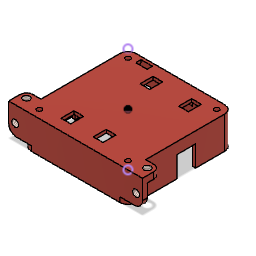
Com Top A (Autodesk Fusion 360 design; units mm, degrees)
Autodesk Fusion 360 part; units mm, degrees
sketch "Sketch17" plane through (0, 0, 0) normal (0, 1, 0) x (1, 0, 0)
  line L0 (-32.5, 32.5) -> (32.5, 32.5)
  line L1 (32.5, 32.5) -> (32.5, -32.5)
  line L2 (32.5, -32.5) -> (-32.5, -32.5)
  line L3 (-32.5, -32.5) -> (-32.5, 32.5)
  line L4 (-32.5, 32.5) -> (32.5, -32.5) construction
  line L5 (32.5, 32.5) -> (-32.5, -32.5) construction
  dimension "d63" = 65
  dimension "d64" = 65
  constraint horizontal L0
  constraint perpendicular L0 L1
  constraint parallel L0 L2
  constraint parallel L1 L3
  constraint coincident L4 origin
  constraint coincident L5 origin
  measures "d63" distance of L1.end L2.end
  measures "d64" distance of L0.end L1.end
extrude "Extrude19" add sketch "Sketch17" along normal blind 2 makes body 1
sketch "Sketch18" plane through (0, 2, 0) normal (0, 1, 0) x (-1, 0, 0)
  line L0 (-32.5, 32.5) -> (-32.5, -32.5)
  line L1 (-32.5, -32.5) -> (32.5, -32.5)
sketch "Sketch20" plane through (0, 0, 0) normal (0, -1, 0) x (1, 0, 0)
  line L0 (32.5, 32.5) -> (-32.5, 32.5)
  line L1 (-32.5, 32.5) -> (-32.5, -32.5)
  line L2 (-32.5, -32.5) -> (32.5, -32.5)
  line L3 (32.5, -32.5) -> (32.5, 32.5)
  line L4 (30.75, -30.75) -> (-30.75, -30.75)
  line L5 (-30.75, -30.75) -> (-30.75, 30.75)
  line L6 (-30.75, 30.75) -> (30.75, 30.75)
  line L7 (30.75, 30.75) -> (30.75, -30.75)
  line L8 (30.75, -30.75) -> (-30.75, 30.75) construction
  line L9 (-30.75, -30.75) -> (30.75, 30.75) construction
  line L10 (-32.5, 22.7576) -> (-30.75, 22.7576)
  line L11 (-30.75, 22.7576) -> (-30.75, 2.2148)
  line L12 (-30.75, 2.2148) -> (-32.5, 2.2148)
  line L13 (-32.5, 2.2148) -> (-32.5, 22.7576)
  line L14 (-32.5, -3.5662) -> (-30.75, -3.5662)
  line L15 (-30.75, -3.5662) -> (-30.75, -14.3569)
  line L16 (-30.75, -14.3569) -> (-32.5, -14.3569)
  line L17 (-32.5, -14.3569) -> (-32.5, -3.5662)
  line L18 (-22.4493, -30.75) -> (-15.7732, -30.75)
  line L19 (-15.7732, -30.75) -> (-15.7732, -32.5)
  line L20 (-15.7732, -32.5) -> (-22.4493, -32.5)
  line L21 (-22.4493, -32.5) -> (-22.4493, -30.75)
  line L22 (-3.0358, -30.75) -> (9.2826, -30.75)
  line L23 (9.2826, -30.75) -> (9.2826, -32.5)
  line L24 (9.2826, -32.5) -> (-3.0358, -32.5)
  line L25 (-3.0358, -32.5) -> (-3.0358, -30.75)
  line L26 (30.75, 1.1041) -> (32.5, 1.1041)
  line L27 (32.5, 1.1041) -> (32.5, -8.4005)
  line L28 (32.5, -8.4005) -> (30.75, -8.4005)
  line L29 (30.75, -8.4005) -> (30.75, 1.1041)
  dimension "d69" = 61.5
  dimension "d70" = 61.5
  constraint horizontal L4
  constraint perpendicular L4 L5
  constraint parallel L4 L6
  constraint parallel L5 L7
  constraint coincident L8 origin
  constraint coincident L9 origin
  constraint horizontal L10
  constraint vertical L11
  constraint horizontal L12
  constraint vertical L13
  constraint coincident L5 L11.end
  constraint coincident L1 L10.start
  constraint horizontal L14
  constraint vertical L15
  constraint horizontal L16
  constraint vertical L17
  constraint coincident L5 L15.end
  constraint coincident L1 L14.start
  constraint horizontal L18
  constraint vertical L19
  constraint horizontal L20
  constraint vertical L21
  constraint coincident L2 L19.end
  constraint coincident L4 L18.start
  constraint horizontal L22
  constraint vertical L23
  constraint horizontal L24
  constraint vertical L25
  constraint coincident L2 L23.end
  constraint coincident L4 L22.start
  constraint horizontal L26
  constraint vertical L27
  constraint horizontal L28
  constraint vertical L29
  constraint coincident L3 L27.end
  constraint coincident L7 L26.start
  measures "d69" distance of L5.end L6.end
  measures "d70" distance of L4.end L5.end
extrude "Extrude20" add sketch "Sketch20" along normal blind 25 contours L0 L1 L3 L5 L6 L7 L10 L26 | L2 L3 L4 L7 L23 L28 | L1 L5 L12 L14 | L1 L2 L4 L5 L16 L21 | L2 L4 L19 L25 bodies 1
extrude "Extrude21" add 1 faces at (32.5, -7.6667, 22.0347) along direction (1, 0, 0) blind 1 on bodies 1 bodies 1
extrude "Extrude22" add 1 faces at (25.4275, -7.6667, -32.5) along direction (0, 0, -1) blind 1 on bodies 1 bodies 1
extrude "Extrude23" add 1 faces at (-32.5, -7.6667, -27.119) along direction (-1, 0, 0) blind 1 on bodies 1 bodies 1
extrude "Extrude24" add 1 faces at (11.1667, -16, 32.5) along direction (0, 0, 1) blind 1 on bodies 1 bodies 1
sketch "Sketch21" plane through (0, 0, 0) normal (0, -1, 0) x (1, 0, 0)
  line L0 (-15.7732, -33.5) -> (-15.7732, -30.75)
  line L1 (-15.7732, -30.75) -> (-3.0358, -30.75)
  line L2 (-3.0358, -30.75) -> (-3.0358, -33.5)
  line L3 (-3.0358, -33.5) -> (9.2826, -33.5)
  line L4 (9.2826, -33.5) -> (9.2826, -30.75)
  line L5 (9.2826, -30.75) -> (30.75, -30.75)
  line L6 (30.75, -30.75) -> (30.75, -8.4005)
  line L7 (30.75, -8.4005) -> (33.5, -8.4005)
  line L8 (33.5, -8.4005) -> (33.5, 1.1041)
  line L9 (33.5, 1.1041) -> (30.75, 1.1041)
  line L10 (30.75, 1.1041) -> (30.75, 30.75)
  line L11 (30.75, 30.75) -> (-30.75, 30.75)
  line L12 (-30.75, 30.75) -> (-30.75, 22.7576)
  line L13 (-30.75, 22.7576) -> (-33.5, 22.7576)
  line L14 (-33.5, 22.7576) -> (-33.5, 2.2148)
  line L15 (-33.5, 2.2148) -> (-30.75, 2.2148)
  line L16 (-30.75, 2.2148) -> (-30.75, -3.5662)
  line L17 (-30.75, -3.5662) -> (-33.5, -3.5662)
  line L18 (-33.5, -3.5662) -> (-33.5, -14.3569)
  line L19 (-33.5, -14.3569) -> (-30.75, -14.3569)
  line L20 (-30.75, -14.3569) -> (-30.75, -30.75)
  line L21 (-30.75, -30.75) -> (-22.4493, -30.75)
  line L22 (-22.4493, -30.75) -> (-22.4493, -33.5)
  line L23 (-22.4493, -33.5) -> (-15.7732, -33.5)
  line L24 (30.75, -30.75) -> (-30.75, -30.75)
  line L25 (-30.75, -30.75) -> (-30.75, 30.75)
  line L26 (-30.75, 30.75) -> (30.75, 30.75)
  line L27 (30.75, 30.75) -> (30.75, -30.75)
  line L28 (30.75, -30.75) -> (-30.75, 30.75) construction
  line L29 (-30.75, -30.75) -> (30.75, 30.75) construction
  constraint horizontal L24
  constraint perpendicular L24 L25
  constraint parallel L24 L26
  constraint parallel L25 L27
  constraint coincident L28 origin
  constraint coincident L29 origin
  constraint coincident L5.end L6.start
extrude "Extrude25" add sketch "Sketch21" along normal blind 23 contours L0 L22 L23 L24 | L2 L3 L4 L24 | L17 L18 L19 L25 | L7 L8 L9 L27 | L13 L14 L15 L25 bodies 1
sketch "Sketch22" plane through (0, 0, 0) normal (0, -1, 0) x (1, 0, 0)
  line L0 (-30.75, -30.75) -> (30.75, -30.75)
  line L1 (30.75, -30.75) -> (30.75, 30.75)
  line L2 (30.75, 30.75) -> (-30.75, 30.75)
  line L3 (-30.75, 30.75) -> (-30.75, -30.75)
  line L4 (30.75, 30.75) -> (24.75, 30.75)
  line L5 (24.75, 30.75) -> (24.75, 24.75)
  line L6 (24.75, 24.75) -> (30.75, 24.75)
  line L7 (30.75, 24.75) -> (30.75, 30.75)
  line L8 (-30.75, 30.75) -> (-24.75, 30.75)
  line L9 (-24.75, 30.75) -> (-24.75, 24.75)
  line L10 (-24.75, 24.75) -> (-30.75, 24.75)
  line L11 (-30.75, 24.75) -> (-30.75, 30.75)
  line L12 (-30.75, -30.75) -> (-24.75, -30.75)
  line L13 (-24.75, -30.75) -> (-24.75, -24.75)
  line L14 (-24.75, -24.75) -> (-30.75, -24.75)
  line L15 (-30.75, -24.75) -> (-30.75, -30.75)
  line L16 (30.75, -30.75) -> (24.75, -30.75)
  line L17 (24.75, -30.75) -> (24.75, -24.75)
  line L18 (24.75, -24.75) -> (30.75, -24.75)
  line L19 (30.75, -24.75) -> (30.75, -30.75)
  dimension "d83" = 6
  dimension "d84" = 6
  dimension "d85" = 6
  dimension "d86" = 6
  dimension "d87" = 6
  dimension "d88" = 6
  dimension "d89" = 6
  dimension "d90" = 6
  constraint horizontal L4
  constraint vertical L5
  constraint horizontal L6
  constraint vertical L7
  constraint coincident L1.end L2.start
  constraint horizontal L8
  constraint vertical L9
  constraint horizontal L10
  constraint vertical L11
  constraint coincident L2.end L3.start
  constraint horizontal L12
  constraint vertical L13
  constraint horizontal L14
  constraint vertical L15
  constraint coincident L0.start L3.end
  constraint horizontal L16
  constraint vertical L17
  constraint horizontal L18
  constraint vertical L19
  constraint coincident L0.end L1.start
  measures "d83" distance of L1.end L4.end
  measures "d84" distance of L1.end L6.end
  measures "d85" distance of L2.end L8.end
  measures "d86" distance of L2.end L10.end
  measures "d87" distance of L0.start L12.end
  measures "d88" distance of L0.start L14.end
  measures "d89" distance of L0.end L16.end
  measures "d90" distance of L0.end L18.end
extrude "Extrude26" add sketch "Sketch22" along normal blind 23.5 contours L0 L3 L12 L13 L14 L15 | L0 L1 L16 L17 L18 L19 | L2 L3 L8 L9 L10 L11 | L1 L2 L4 L5 L6 L7 bodies 1
fillet "Fillet3" radius 4 4 edges at (-24.75, -11.75, 24.75) (24.75, -11.75, 24.75) (-24.75, -11.75, -24.75) (24.75, -11.75, -24.75) on bodies 1
fillet "Fillet4" radius 6 3 edges at (33.5, -11.5, -33.5) (-33.5, -11.5, 33.5) (-33.5, -11.5, -33.5) on bodies 1
fillet "Fillet5" radius 6 1 edges at (33.5, -11.5, 33.5) on bodies 1
extrude "Extrude27" cut 1 faces at (-31.6667, -23, 9.0624) along direction (0, 1, 0) blind 2 on bodies 1 bodies 1
extrude "Extrude28" cut 1 faces at (-32.5833, -23, -10.76) along direction (0, 1, 0) blind 5 on bodies 1 bodies 1
extrude "Extrude29" cut 1 faces at (32.5833, -23, -5.2323) along direction (0, 1, 0) blind 10 on bodies 1 bodies 1
extrude "Extrude30" cut 1 faces at (-17.9986, -23, -32.5833) along direction (0, 1, 0) blind 6 on bodies 1 bodies 1
extrude "Extrude31" cut 1 faces at (-32.5833, -18, -10.76) along direction (0, 1, 0) blind 5 on bodies 1 bodies 1
extrude "Extrude32" cut 1 faces at (-31.6667, -21, 9.0624) along direction (0, 1, 0) blind 2 on bodies 1 bodies 1
sketch "Sketch23" plane through (0, 2, 0) normal (0, 1, 0) x (-1, 0, 0)
  line L0 (27.6499, -33.4994) -> (22.6499, -33.4994)
  line L1 (22.6499, -33.4994) -> (15.6499, -33.4994)
  line L2 (15.6499, -33.4994) -> (15.6499, -27.4994)
  line L3 (15.6499, -27.4994) -> (22.6499, -27.4994)
  line L4 (22.6499, -27.4994) -> (22.6499, -33.4994)
  line L5 (15.6499, -27.4994) -> (22.6499, -27.4994)
  line L6 (22.6499, -27.4994) -> (22.6499, -31.4994)
  line L7 (22.6499, -31.4994) -> (15.6499, -31.4994)
  line L8 (15.6499, -31.4994) -> (15.6499, -27.4994)
  dimension "d123" = 5
  dimension "d124" = 7
  dimension "d125" = 6
  dimension "d126" = 4
  constraint horizontal L0
  constraint horizontal L1
  constraint vertical L2
  constraint horizontal L3
  constraint vertical L4
  constraint horizontal L5
  constraint vertical L6
  constraint horizontal L7
  constraint vertical L8
  measures "d123" distance of L0.start L0.end
  measures "d124" distance of L0.end L1.end
  measures "d125" distance of L0.end L3.end
  measures "d126" distance of L2.end L7.end
extrude "Extrude33" cut sketch "Sketch23" against normal blind 3 contours L2 L3 L4 L5 L6 L7 L8 bodies 1
sketch "Sketch24" plane through (0, 0, -33.5) normal (0, 0, -1) x (-1, 0, 0)
  line L0 (15.7732, -25) -> (15.7732, -17)
  line L1 (15.7732, -17) -> (22.4493, -17)
  line L2 (22.4493, -17) -> (22.4493, -25)
  line L3 (22.4493, -25) -> (27.5, -25)
  line L4 (27.5, -25) -> (27.5, 2)
  line L5 (27.5, 2) -> (-27.5, 2)
  line L6 (-27.5, 2) -> (-27.5, -25)
  line L7 (-27.5, -25) -> (-9.2826, -25)
  line L8 (-9.2826, -25) -> (-9.2826, -23)
  line L9 (-9.2826, -23) -> (3.0358, -23)
  line L10 (3.0358, -23) -> (3.0358, -25)
  line L11 (3.0358, -25) -> (15.7732, -25)
  line L12 (-9.2826, 2) -> (-9.2826, -25)
  line L13 (3.0358, -25) -> (3.0358, 2)
  line L14 (-4.7559, 2) -> (-4.7559, -4)
  line L15 (-9.2826, -4) -> (3.0358, -4)
  line L16 (3.0358, -4) -> (3.0358, -11.5)
  line L17 (3.0358, -11.5) -> (-9.2826, -11.5)
  line L18 (-9.2826, -11.5) -> (-9.2826, -4)
  dimension "d129" = 6
  constraint coincident L5 L12.start
  constraint coincident L7.end L8.start
  constraint perpendicular L5 L12
  constraint coincident L10.end L11.start
  constraint coincident L5 L13.end
  constraint perpendicular L5 L13
  constraint coincident L5 L14.start
  constraint perpendicular L5 L14
  constraint horizontal L15
  constraint vertical L16
  constraint horizontal L17
  constraint vertical L18
  constraint midpoint L13 L16.end
  constraint coincident L12 L15.start
  measures "d129" distance of L14.start L14.end
extrude "Extrude34" cut sketch "Sketch24" against normal blind 10 contours L12 L13 L15 L16 L17 L18 bodies 1
extrude "Extrude35" add 1 faces at (1.0703, -23, -31.6667) along direction (0, -1, 0) blind 2 on bodies 1 bodies 1
delete_face "DeleteFace1" 1 faces at (28.0703, -7, 33.4728) on bodies 1
delete_face "DeleteFace2" 1 faces at (-28.0703, -16, 33.4728) on bodies 1
sketch "Sketch25" plane through (-33.5, 0, 0) normal (-1, 0, 0) x (0, 0, 1)
  line L0 (33.5, 2) -> (-27.5, 2)
  line L1 (-27.5, 2) -> (-27.5, -25)
  line L2 (-27.5, -25) -> (-14.3569, -25)
  line L3 (-14.3569, -25) -> (-14.3569, -13)
  line L4 (-14.3569, -13) -> (-3.5662, -13)
  line L5 (-3.5662, -13) -> (-3.5662, -25)
  line L6 (-3.5662, -25) -> (2.2148, -25)
  line L7 (2.2148, -25) -> (2.2148, -19)
  line L8 (2.2148, -19) -> (22.7576, -19)
  line L9 (22.7576, -19) -> (22.7576, -25)
  line L10 (22.7576, -25) -> (33.5, -25)
  line L11 (33.5, -25) -> (33.5, 2)
  line L12 (33.5, 2) -> (29.5, 2)
  line L13 (29.5, 2) -> (29.5, -25)
  line L14 (29.5, -25) -> (33.5, -25)
  line L15 (33.5, -25) -> (33.5, 2)
  dimension "d134" = 4
  constraint horizontal L12
  constraint vertical L13
  constraint horizontal L14
  constraint vertical L15
  constraint coincident L0.start L11.end
  measures "d134" distance of L0.start L12.end
extrude "Extrude36" add sketch "Sketch25" along normal blind 8 contours L0 L10 L11 L12 L13 L14 L15 bodies 1
sketch "Sketch26" plane through (33.5, 0, 0) normal (1, 0, 0) x (0, 0, -1)
  line L0 (-33.5, -25) -> (-1.1041, -25)
  line L1 (-1.1041, -25) -> (-1.1041, -13)
  line L2 (-1.1041, -13) -> (8.4005, -13)
  line L3 (8.4005, -13) -> (8.4005, -25)
  line L4 (8.4005, -25) -> (27.5, -25)
  line L5 (27.5, -25) -> (27.5, 2)
  line L6 (27.5, 2) -> (-33.5, 2)
  line L7 (-33.5, 2) -> (-33.5, -25)
  line L8 (-33.5, 2) -> (-29.5, 2)
  line L9 (-29.5, 2) -> (-29.5, -25)
  line L10 (-29.5, -25) -> (-33.5, -25)
  line L11 (-33.5, -25) -> (-33.5, 2)
  dimension "d137" = 4
  constraint horizontal L8
  constraint vertical L9
  constraint horizontal L10
  constraint vertical L11
  constraint coincident L6.end L7.start
  measures "d137" distance of L6.end L8.end
extrude "Extrude37" add sketch "Sketch26" along normal blind 8 contours L0 L6 L7 L8 L9 L10 L11 bodies 1
sketch "Sketch27" plane through (0, 0, 29.5) normal (0, 0, -1) x (-1, 0, 0)
  line L0 (33.5, 2) -> (33.5, -25)
  line L1 (33.5, -25) -> (41.5, -25)
  line L2 (41.5, -25) -> (41.5, 2)
  line L3 (41.5, 2) -> (33.5, 2)
  line L4 (37.5, 2) -> (37.5, -25)
  line L5 (37.5, 2) -> (37.5, -8)
  dimension "d140" = 10
  constraint midpoint L3 L4.start
  constraint midpoint L1 L4.end
  constraint perpendicular L3 L5
  measures "d140" distance of L4.start L5.end
hole "Hole6" at (-37.5, -8, 29.5) direction (0, 0, 1) diameter 4.234 depth 13 tip angle 118 bodies 1
thread "Thread6" "ISO Metric profile 5.0 M5x0.8 6H" major diameter 5.12 minor diameter 4.234 pitch 0.8 angle 60 resizes the face on face at (-37.2892, -5.8935, 32.1667) on bodies 1
sketch "Sketch28" plane through (0, 0, 29.5) normal (0, 0, -1) x (-1, 0, 0)
  line L0 (-33.5, -25) -> (-33.5, 2)
  line L1 (-33.5, 2) -> (-41.5, 2)
  line L2 (-41.5, 2) -> (-41.5, -25)
  line L3 (-41.5, -25) -> (-33.5, -25)
  line L4 (-37.5, 2) -> (-37.5, -8)
  dimension "d144" = 10
  constraint midpoint L1 L4.start
  constraint perpendicular L1 L4
  measures "d144" distance of L4.start L4.end
hole "Hole7" at (37.5, -8, 29.5) direction (0, 0, 1) diameter 4.234 depth 12 tip angle 118 bodies 1
thread "Thread7" "ISO Metric profile 5.0 M5x0.8 6H" major diameter 5.12 minor diameter 4.234 pitch 0.8 angle 60 resizes the face on face at (35.5703, -8.8707, 30.8333) on bodies 1
sketch "Sketch29" plane through (0, -25, 0) normal (0, -1, 0) x (1, 0, 0)
  line L0 (-33.5, 29.5) -> (-33.5, 22.7576)
  line L1 (-33.5, 22.7576) -> (-30.75, 22.7576)
  line L2 (-30.75, 22.7576) -> (-30.75, 30.75)
  line L3 (-30.75, 30.75) -> (30.75, 30.75)
  line L4 (30.75, 30.75) -> (30.75, 1.1041)
  line L5 (30.75, 1.1041) -> (33.5, 1.1041)
  line L6 (33.5, 1.1041) -> (33.5, 29.5)
  line L7 (33.5, 29.5) -> (41.5, 29.5)
  line L8 (41.5, 29.5) -> (41.5, 33.5)
  line L9 (41.5, 33.5) -> (-41.5, 33.5)
  line L10 (-41.5, 33.5) -> (-41.5, 29.5)
  line L11 (-41.5, 29.5) -> (-33.5, 29.5)
  line L12 (-33.5, 29.5) -> (-33.5, 33.5)
  line L13 (33.5, 29.5) -> (33.5, 33.5)
  constraint coincident L0.start L11.end
  constraint coincident L9 L12.end
  constraint perpendicular L9 L12
  constraint coincident L6.end L7.start
  constraint coincident L9 L13.end
  constraint perpendicular L9 L13
extrude "Extrude38" cut sketch "Sketch29" against normal blind 10 contours L9 L10 L11 L12 | L7 L8 L9 L13 bodies 1
fillet "Fillet6" radius 6 2 edges at (33.5, -20, 33.5) (-33.5, -20, 33.5) on bodies 1
fillet "Fillet7" radius 5 1 edges at (41.5, -15, 31.5) on bodies 1
fillet "Fillet8" radius 5 1 edges at (-41.5, -15, 31.5) on bodies 1
sketch "Sketch30" plane through (0, 0, 0) normal (0, -1, 0) x (1, 0, 0)
  line L0 (-15.6499, -27.4994) -> (-15.6499, -30.75)
  line L1 (-15.6499, -30.75) -> (24.75, -30.75)
  line L2 (24.75, -30.75) -> (24.75, -28.75)
  arc A0 (28.75, -24.75) -> (24.75, -28.75) centre (28.75, -28.75) ccw
  line L3 (28.75, -24.75) -> (30.75, -24.75)
  line L4 (30.75, -24.75) -> (30.75, 24.75)
  line L5 (30.75, 24.75) -> (28.75, 24.75)
  arc A1 (24.75, 28.75) -> (28.75, 24.75) centre (28.75, 28.75) ccw
  line L6 (24.75, 28.75) -> (24.75, 30.75)
  line L7 (24.75, 30.75) -> (-24.75, 30.75)
  line L8 (-24.75, 30.75) -> (-24.75, 28.75)
  arc A2 (-28.75, 24.75) -> (-24.75, 28.75) centre (-28.75, 28.75) ccw
  line L9 (-28.75, 24.75) -> (-30.75, 24.75)
  line L10 (-30.75, 24.75) -> (-30.75, -24.75)
  line L11 (-30.75, -24.75) -> (-28.75, -24.75)
  arc A3 (-24.75, -28.75) -> (-28.75, -24.75) centre (-28.75, -28.75) ccw
  line L12 (-24.75, -28.75) -> (-24.75, -30.75)
  line L13 (-24.75, -30.75) -> (-22.6499, -30.75)
  line L14 (-22.6499, -30.75) -> (-22.6499, -27.4994)
  line L15 (-22.6499, -27.4994) -> (-15.6499, -27.4994)
  line L16 (14, -17.5) -> (-14, -17.5)
  line L17 (-14, -17.5) -> (-14, 17.5)
  line L18 (-14, 17.5) -> (14, 17.5)
  line L19 (14, 17.5) -> (14, -17.5)
  line L20 (14, -17.5) -> (-14, 17.5) construction
  line L21 (-14, -17.5) -> (14, 17.5) construction
  line L22 (14, 17.5) -> (20, 17.5)
  line L23 (20, 17.5) -> (20, 25.5)
  line L24 (20, 25.5) -> (14, 25.5)
  line L25 (14, 25.5) -> (14, 17.5)
  line L26 (14, -17.5) -> (20, -17.5)
  line L27 (20, -17.5) -> (20, -25.5)
  line L28 (20, -25.5) -> (14, -25.5)
  line L29 (14, -25.5) -> (14, -17.5)
  line L30 (-14, -17.5) -> (-20, -17.5)
  line L31 (-20, -17.5) -> (-20, -25.5)
  line L32 (-20, -25.5) -> (-14, -25.5)
  line L33 (-14, -25.5) -> (-14, -17.5)
  line L34 (-14, 17.5) -> (-20, 17.5)
  line L35 (-20, 17.5) -> (-20, 25.5)
  line L36 (-20, 25.5) -> (-14, 25.5)
  line L37 (-14, 25.5) -> (-14, 17.5)
  dimension "d156" = 28
  dimension "d157" = 35
  dimension "d158" = 6
  dimension "d159" = 8
  dimension "d160" = 6
  dimension "d161" = 8
  dimension "d162" = 6
  dimension "d163" = 8
  dimension "d164" = 6
  dimension "d165" = 8
  constraint horizontal L16
  constraint perpendicular L16 L17
  constraint parallel L16 L18
  constraint parallel L17 L19
  constraint coincident L20 origin
  constraint coincident L21 origin
  constraint horizontal L22
  constraint vertical L23
  constraint horizontal L24
  constraint vertical L25
  constraint horizontal L26
  constraint vertical L27
  constraint horizontal L28
  constraint vertical L29
  constraint horizontal L30
  constraint vertical L31
  constraint horizontal L32
  constraint vertical L33
  constraint horizontal L34
  constraint vertical L35
  constraint horizontal L36
  constraint vertical L37
  measures "d156" distance of L17.end L18.end
  measures "d157" distance of L16.end L17.end
  measures "d158" distance of L18.end L22.end
  measures "d159" distance of L18.end L24.end
  measures "d160" distance of L16.start L26.end
  measures "d161" distance of L16.start L28.end
  measures "d162" distance of L16.end L30.end
  measures "d163" distance of L16.end L32.end
  measures "d164" distance of L17.end L34.end
  measures "d165" distance of L17.end L36.end
extrude "Extrude39" cut sketch "Sketch30" against normal blind 35 contours L30 L31 L32 L33 | L34 L35 L36 L37 | L22 L23 L24 L25 | L26 L27 L28 L29 bodies 1
extrude "Extrude40" add 1 faces at (-20.3166, -1, -31.2496) along direction (0, 1, 0) blind 3 on bodies 1 bodies 1
delete_face "DeleteFace3" 1 faces at (-33.3331, -12.6667, 28.9052) on bodies 1
delete_face "DeleteFace4" 1 faces at (33.3331, -12.6667, 28.9052) on bodies 1
sketch "Sketch32" plane through (0, 2, 0) normal (0, 1, 0) x (-1, 0, 0)
  line L0 (20, 25.5) -> (20, 17.5)
  line L1 (20, 17.5) -> (14, 17.5)
  line L2 (14, 17.5) -> (14, 25.5)
  line L3 (14, 25.5) -> (20, 25.5)
  line L4 (-14, 17.5) -> (-20, 17.5)
  line L5 (-20, 17.5) -> (-20, 25.5)
  line L6 (-20, 25.5) -> (-14, 25.5)
  line L7 (-14, 25.5) -> (-14, 17.5)
  line L8 (14, -17.5) -> (20, -17.5)
  line L9 (20, -17.5) -> (20, -25.5)
  line L10 (20, -25.5) -> (14, -25.5)
  line L11 (14, -25.5) -> (14, -17.5)
  line L12 (-20, -25.5) -> (-20, -17.5)
  line L13 (-20, -17.5) -> (-14, -17.5)
  line L14 (-14, -17.5) -> (-14, -25.5)
  line L15 (-14, -25.5) -> (-20, -25.5)
  line L16 (22.6499, -27.4994) -> (22.6499, -30.75)
  line L17 (22.6499, -30.75) -> (15.6499, -30.75)
  line L18 (15.6499, -30.75) -> (15.6499, -27.4994)
  line L19 (15.6499, -27.4994) -> (22.6499, -27.4994)
  line L20 (41.5, 33.5) -> (-41.5, 33.5)
  line L21 (-41.5, 33.5) -> (-41.5, 29.5)
  line L22 (-41.5, 29.5) -> (-33.5, 29.5)
  line L23 (-33.5, 29.5) -> (-33.5, -27.5)
  arc A0 (-33.5, -27.5) -> (-27.5, -33.5) centre (-27.5, -27.5) ccw
  line L24 (-27.5, -33.5) -> (27.5, -33.5)
  arc A1 (27.5, -33.5) -> (33.5, -27.5) centre (27.5, -27.5) ccw
  line L25 (33.5, -27.5) -> (33.5, 29.5)
  line L26 (33.5, 29.5) -> (41.5, 29.5)
  line L27 (41.5, 29.5) -> (41.5, 33.5)
  line L28 (33.5, 29.5) -> (41.5, 29.5)
  line L29 (41.5, 29.5) -> (41.5, 21.5)
  line L30 (41.5, 21.5) -> (33.5, 21.5)
  line L31 (33.5, 21.5) -> (33.5, 29.5)
  line L32 (-33.5, 29.5) -> (-41.5, 29.5)
  line L33 (-41.5, 29.5) -> (-41.5, 21.5)
  line L34 (-41.5, 21.5) -> (-33.5, 21.5)
  line L35 (-33.5, 21.5) -> (-33.5, 29.5)
  dimension "d170" = 8
  dimension "d171" = 8
  dimension "d172" = 8
  constraint horizontal L28
  constraint vertical L29
  constraint horizontal L30
  constraint vertical L31
  constraint coincident L25.end L26.start
  constraint horizontal L32
  constraint vertical L33
  constraint horizontal L34
  constraint vertical L35
  constraint coincident L22.end L23.start
  measures "d170" distance of L25.end L30.end
  measures "d171" distance of L22.end L21.end
  measures "d172" distance of L22.end L34.end
extrude "Extrude41" add sketch "Sketch32" against normal blind 4 contours L25 L26 L28 L29 L30 L31 | L22 L23 L32 L33 L34 L35 bodies 1
sketch "Sketch33" plane through (0, -2, 0) normal (0, -1, 0) x (1, 0, 0)
  line L0 (33.5, 29.5) -> (33.5, 21.5)
  line L1 (33.5, 21.5) -> (41.5, 21.5)
  line L2 (41.5, 21.5) -> (41.5, 29.5)
  line L3 (41.5, 29.5) -> (33.5, 29.5)
  line L4 (37.5, 25.5) -> (37.5, 21.5)
  constraint midpoint L1 L4.end
  constraint perpendicular L1 L4
hole "Hole8" at (37.5, -2, 25.5) direction (0, 1, 0) diameter 4.234 depth 8 tip angle 118 bodies 1
thread "Thread8" "ISO Metric profile 5.0 M5x0.8 6H" major diameter 5.12 minor diameter 4.234 pitch 0.8 angle 60 resizes the face on face at (35.7217, -0.6667, 24.3514) on bodies 1
sketch "Sketch34" plane through (0, -2, 0) normal (0, -1, 0) x (1, 0, 0)
  line L0 (-41.5, 21.5) -> (-33.5, 21.5)
  line L1 (-33.5, 21.5) -> (-33.5, 29.5)
  line L2 (-33.5, 29.5) -> (-41.5, 29.5)
  line L3 (-41.5, 29.5) -> (-41.5, 21.5)
  line L4 (-37.5, 25.5) -> (-37.5, 21.5)
  constraint midpoint L0 L4.end
  constraint perpendicular L0 L4
hole "Hole9" at (-37.5, -2, 25.5) direction (0, 1, 0) diameter 4.234 depth 7 tip angle 118 bodies 1
thread "Thread9" "ISO Metric profile 5.0 M5x0.8 6H" major diameter 5.12 minor diameter 4.234 pitch 0.8 angle 60 resizes the face on face at (-36.3961, -0.6667, 27.3064) on bodies 1
fillet "Fillet9" radius 4 2 edges at (41.5, 0, 21.5) (-41.5, 0, 21.5) on bodies 1
fillet "Fillet10" radius 4 1 edges at (-33.5, -20, 33.5) on bodies 1
fillet "Fillet11" radius 4 1 edges at (33.5, -20, 33.5) on bodies 1
delete_face "DeleteFace5" 1 faces at (33.4955, -18.3333, 29.6903) on bodies 1
delete_face "DeleteFace6" 1 faces at (-33.4955, -18.3333, 29.6903) on bodies 1
delete_face "DeleteFace7" 1 faces at (31.209, -7, -32.2163) on bodies 1
delete_face "DeleteFace8" 1 faces at (-33.4728, -16, -28.0703) on bodies 1
extrude "Extrude42" cut 1 faces at (25.4275, -11.5, -33.5) along direction (0, 0, 1) blind 1 on bodies 1 bodies 1
extrude "Extrude43" cut 1 faces at (33.5, -12, -24.4668) along direction (-1, 0, 0) blind 1 on bodies 1 bodies 1
extrude "Extrude44" cut 1 faces at (10.5, -21.6667, 33.5) along direction (0, 0, -1) blind 1 on bodies 1 bodies 1
extrude "Extrude45" cut 1 faces at (-33.5, -3, -4.8554) along direction (1, 0, 0) blind 1 on bodies 1 bodies 1
fillet "Fillet12" radius 5 4 edges at (32.5, -11.5, -32.5) (-32.5, -11.5, -32.5) (32.5, -20, 32.5) (-32.5, -20, 32.5) on bodies 1
extrude "Extrude46" cut 1 faces at (-31.9167, -13, -10.76) along direction (0, 1, 0) blind 4 on bodies 1 bodies 1
extrude "Extrude47" cut 1 faces at (-31.9167, -19, 15.91) along direction (0, 1, 0) blind 4 on bodies 1 bodies 1
extrude "Extrude48" cut 4 faces at (-30.0833, -23.5, 26.75) (-30.0833, -23.5, -26.75) (26.75, -23.5, -30.0833) (30.0833, -23.5, 26.75) along direction (0, 1, 0) blind 4 on bodies 1 bodies 1
extrude "Extrude49" cut 1 faces at (31.9167, -13, -5.2323) along direction (0, 1, 0) blind 4 on bodies 1 bodies 1
extrude "Extrude50" cut 1 faces at (-20.2239, -17, -31.9167) along direction (0, 1, 0) blind 4 on bodies 1 bodies 1
extrude "Extrude51" cut 4 faces at (-31.3333, -25, -24.2023) (14.1589, -25, -31.3333) (-9.1667, -25, 31.3333) (-31.9167, -25, -1.6392) along direction (0, 1, 0) blind 4 on bodies 1 bodies 1
extrude "Extrude52" cut 1 faces at (5.1765, -4, -31.9167) along direction (0, 1, 0) blind 3 on bodies 1 bodies 1
delete_face "DeleteFace9" 1 faces at (24.7681, -6.5, -28.3698) on bodies 1
delete_face "DeleteFace10" 1 faces at (24.7681, -6.5, 28.3698) on bodies 1
delete_face "DeleteFace11" 1 faces at (-28.3698, -6.5, -24.7681) on bodies 1
delete_face "DeleteFace12" 1 faces at (-28.3698, -6.5, 24.7681) on bodies 1
extrude "Extrude53" cut 1 faces at (5.1765, -1, -31.9167) along direction (0, 1, 0) blind 0.5 on bodies 1 bodies 1
extrude "Extrude54" add 1 faces at (1.0703, -11.5, -31.9167) along direction (0, 1, 0) blind 0.5 on bodies 1 bodies 1
extrude "Extrude55" cut 4 faces at (26.75, -19.5, 28.75) (-28.75, -19.5, 26.75) (-28.75, -19.5, -26.75) (26.75, -19.5, -28.75) along direction (0, 1, 0) blind 0.5 on bodies 1 bodies 1
sketch "Sketch35" plane through (0, 2, 0) normal (0, 1, 0) x (-1, 0, 0)
  line L0 (22.6499, -27.4994) -> (22.6499, -30.75)
  line L1 (22.6499, -30.75) -> (15.6499, -30.75)
  line L2 (15.6499, -30.75) -> (15.6499, -27.4994)
  line L3 (15.6499, -27.4994) -> (22.6499, -27.4994)
  line L4 (-20, -25.5) -> (-20, -17.5)
  line L5 (-20, -17.5) -> (-14, -17.5)
  line L6 (-14, -17.5) -> (-14, -25.5)
  line L7 (-14, -25.5) -> (-20, -25.5)
  line L8 (14, -17.5) -> (20, -17.5)
  line L9 (20, -17.5) -> (20, -25.5)
  line L10 (20, -25.5) -> (14, -25.5)
  line L11 (14, -25.5) -> (14, -17.5)
  line L12 (-14, 17.5) -> (-20, 17.5)
  line L13 (-20, 17.5) -> (-20, 25.5)
  line L14 (-20, 25.5) -> (-14, 25.5)
  line L15 (-14, 25.5) -> (-14, 17.5)
  line L16 (20, 25.5) -> (20, 17.5)
  line L17 (20, 17.5) -> (14, 17.5)
  line L18 (14, 17.5) -> (14, 25.5)
  line L19 (14, 25.5) -> (20, 25.5)
  circle A0 centre (-37.5, 25.5) radius 2.117
  circle A1 centre (37.5, 25.5) radius 2.117
  arc A2 (27.5, -32.5) -> (32.5, -27.5) centre (27.5, -27.5) ccw
  line L20 (32.5, -27.5) -> (32.5, 21.5)
  line L21 (32.5, 21.5) -> (37.5, 21.5)
  arc A3 (37.5, 21.5) -> (41.5, 25.5) centre (37.5, 25.5) ccw
  line L22 (41.5, 25.5) -> (41.5, 32.5)
  line L23 (41.5, 32.5) -> (-41.5, 32.5)
  line L24 (-41.5, 32.5) -> (-41.5, 25.5)
  arc A4 (-41.5, 25.5) -> (-37.5, 21.5) centre (-37.5, 25.5) ccw
  line L25 (-37.5, 21.5) -> (-32.5, 21.5)
  line L26 (-32.5, 21.5) -> (-32.5, -27.5)
  arc A5 (-32.5, -27.5) -> (-27.5, -32.5) centre (-27.5, -27.5) ccw
  line L27 (-27.5, -32.5) -> (27.5, -32.5)
  line L28 (27.5, -27.5) -> (-27.5, -27.5)
  line L29 (-27.5, -27.5) -> (-27.5, 27.5)
  line L30 (-27.5, 27.5) -> (27.5, 27.5)
  line L31 (27.5, 27.5) -> (27.5, -27.5)
  line L32 (27.5, -27.5) -> (-27.5, 27.5) construction
  line L33 (-27.5, -27.5) -> (27.5, 27.5) construction
  dimension "d217" = 55
  dimension "d218" = 55
  constraint horizontal L28
  constraint perpendicular L28 L29
  constraint parallel L28 L30
  constraint parallel L29 L31
  constraint coincident L32 origin
  constraint coincident L33 origin
  measures "d217" distance of L29.end L30.end
  measures "d218" distance of A5.centre L29.end
hole "Hole10" at (-27.5, 2, 27.5) at (-27.5, 2, -27.5) at (27.5, 2, -27.5) at (27.5, 2, 27.5) direction (0, -1, 0) diameter 3 depth 34.375 tip angle 118 bodies 1
fillet "Fillet13" radius 4 4 edges at (24.75, -9.5, -24.75) (-24.75, -9.5, -24.75) (-24.75, -9.5, 24.75) (24.75, -9.5, 24.75) on bodies 1
extrude "Extrusion56" cut 4 faces at (-31.3333, -21, -24.2023) (-31.9167, -21, -1.6392) (-9.1667, -21, 31.3333) (14.1589, -21, -31.3333) along direction (0, 1, 0) blind 3 on bodies 1 bodies 1
extrude "Extrusion57" cut 4 faces at (-30.1653, -19, -27.704) (-30.1653, -19, 27.704) (30.1653, -19, 27.704) (30.1653, -19, -27.704) along direction (0, 1, 0) blind 3 on bodies 1 bodies 1
extrude "Extrusion58" add 1 faces at (1.0703, -11, -31.9167) along direction (0, 1, 0) blind 4 on bodies 1 bodies 1
extrude "Extrusion59" cut 1 faces at (5.1765, -0.5, -31.9167) along direction (0, 1, 0) blind 0.5 on bodies 1 bodies 1
extrude "Extrusion60" cut 1 faces at (31.9167, -12, -8.4005) along direction (0, 0, -1) blind 1 on bodies 1 bodies 1
extrude "Extrusion61" cut 1 faces at (31.9167, -9, -5.899) along direction (0, 1, 0) blind 4 on bodies 1 bodies 1
extrude "Extrusion62" cut 1 faces at (31.3333, -9.3333, 1.1041) along direction (0, 0, 1) blind 1 on bodies 1 bodies 1
extrude "Extrusion63" cut 1 faces at (-31.9167, -15, 15.91) along direction (0, 1, 0) blind 1.5 on bodies 1 bodies 1
extrude "Extrusion64" cut 1 faces at (-31.9167, -15, 22.7576) along direction (0, 0, 1) blind 1 on bodies 1 bodies 1
extrude "Extrusion65" cut 1 faces at (-31.9167, -9, -10.76) along direction (0, 1, 0) blind 3 on bodies 1 bodies 1
sketch "Skizze36" plane through (0, -13.5, 0) normal (0, -1, 0) x (1, 0, 0)
  line L0 (-32.5, 23.7576) -> (-32.5, 2.2148)
  line L1 (-32.5, 2.2148) -> (-30.75, 2.2148)
  line L2 (-30.75, 2.2148) -> (-30.75, 23.7576)
  line L3 (-30.75, 23.7576) -> (-32.5, 23.7576)
  line L4 (-30.75, 10.4862) -> (-32.5, 10.4862)
  line L5 (-32.5, 10.4862) -> (-32.5, 15.4862)
  line L6 (-32.5, 15.4862) -> (-30.75, 15.4862)
  line L7 (-30.75, 15.4862) -> (-30.75, 10.4862)
  line L8 (-30.75, 10.4862) -> (-32.5, 15.4862) construction
  line L9 (-32.5, 10.4862) -> (-30.75, 15.4862) construction
  point P0 (-31.625, 12.9862)
  dimension "d246" = 5
  constraint horizontal L4
  constraint perpendicular L4 L5
  constraint parallel L4 L6
  constraint parallel L5 L7
  constraint coincident L8 P0
  constraint coincident L9 P0
  measures "d246" distance of L4.end L5.end
extrude "Extrusion66" add sketch "Skizze36" along normal blind 4 contours L0 L2 L4 L5 L6 L7 bodies 1
extrude "Extrude67" cut 4 faces at (30.1653, -16, 27.704) (30.1653, -16, -27.704) (-30.1653, -16, -27.704) (-30.1653, -16, 27.704) along direction (0, 1, 0) blind 3 on bodies 1 bodies 1
move_face "OffsetFaces1" offset -10 1 faces at (14, 0.6667, 22.8333) on bodies 1
move_face "OffsetFaces2" offset 10 1 faces at (20, 1.3333, 22.8333) on bodies 1
move_face "OffsetFaces3" offset -4 1 faces at (-14, 1.3333, 20.1667) on bodies 1
move_face "OffsetFaces4" offset 4 1 faces at (-20, 0.6667, 20.1667) on bodies 1
move_face "OffsetFaces5" offset -10 1 faces at (-14, 0.6667, -22.8333) on bodies 1
move_face "OffsetFaces6" offset 10 1 faces at (-20, 1.3333, -22.8333) on bodies 1
sketch "Sketch37" plane through (0, -6, 0) normal (0, -1, 0) x (1, 0, 0)
  line L0 (-32.5, -3.5662) -> (-32.5, -14.3569)
  line L1 (-32.5, -14.3569) -> (-30.75, -14.3569)
  line L2 (-30.75, -14.3569) -> (-30.75, -3.5662)
  line L3 (-30.75, -3.5662) -> (-32.5, -3.5662)
  line L4 (-32.5, -3.6173) -> (-32.3, -3.6173)
  line L5 (-32.3, -3.6173) -> (-32.3, -14.3)
  line L6 (-32.3, -14.3) -> (-32.5, -14.3)
  line L7 (-32.5, -14.3) -> (-32.5, -3.6173)
  dimension "d257" = 0.2
  constraint horizontal L4
  constraint vertical L5
  constraint horizontal L6
  constraint vertical L7
  constraint coincident L0 L4.start
  measures "d257" distance of L4.start L4.end
extrude "Extrude68" add sketch "Sketch37" along normal blind 12 contours L0 L4 L5 L6 L7 bodies 1
sketch "Sketch38" plane through (0, -13.5, 0) normal (0, -1, 0) x (1, 0, 0)
  line L0 (-32.5, 15.4862) -> (-30.75, 15.4862)
  line L1 (-30.75, 15.4862) -> (-30.75, 23.7576)
  line L2 (-30.75, 23.7576) -> (-32.5, 23.7576)
  line L3 (-32.5, 23.7576) -> (-32.5, 15.4862)
  line L4 (-32.5, 23.5798) -> (-32.3, 23.5798)
  line L5 (-32.3, 23.5798) -> (-32.3, 15.6954)
  line L6 (-32.3, 15.6954) -> (-32.5, 15.6954)
  line L7 (-32.5, 15.6954) -> (-32.5, 23.5798)
  dimension "d260" = 0.2
  constraint horizontal L4
  constraint vertical L5
  constraint horizontal L6
  constraint vertical L7
  constraint coincident L3 L4.start
  measures "d260" distance of L4.start L4.end
extrude "Extrude69" add sketch "Sketch38" along normal blind 4.5 contours L3 L4 L5 L6 L7 bodies 1
sketch "Sketch39" plane through (0, -13.5, 0) normal (0, -1, 0) x (1, 0, 0)
  line L0 (-30.75, 10.4862) -> (-32.5, 10.4862)
  line L1 (-32.5, 10.4862) -> (-32.5, 2.2148)
  line L2 (-32.5, 2.2148) -> (-30.75, 2.2148)
  line L3 (-30.75, 2.2148) -> (-30.75, 10.4862)
  line L4 (-32.5, 10.3766) -> (-32.3, 10.3766)
  line L5 (-32.3, 10.3766) -> (-32.3, 2.4209)
  line L6 (-32.3, 2.4209) -> (-32.5, 2.4209)
  line L7 (-32.5, 2.4209) -> (-32.5, 10.3766)
  dimension "d263" = 0.2
  constraint horizontal L4
  constraint vertical L5
  constraint horizontal L6
  constraint vertical L7
  constraint coincident L1 L4.start
  measures "d263" distance of L4.start L4.end
extrude "Extrude70" add sketch "Sketch39" along normal blind 4.5 contours L1 L4 L5 L6 L7 bodies 1
extrude "Extrude71" cut 1 faces at (-32.4333, -10, -3.6173) along direction (0, 0, -1) blind 0.1 on bodies 1 bodies 1
extrude "Extrude72" cut 1 faces at (-32.3667, -10, -14.3) along direction (0, 0, 1) blind 0.1 on bodies 1 bodies 1
extrude "Extrude73" add 1 faces at (-32.3, -15, 20.9517) along direction (1, 0, 0) blind 0.2 on bodies 1 bodies 1
extrude "Extrude74" add 1 faces at (-32.3, -15, 7.7247) along direction (1, 0, 0) blind 0.2 on bodies 1 bodies 1
extrude "Extrude75" add 1 faces at (-32.3, -10, -7.2115) along direction (1, 0, 0) blind 0.2 on bodies 1 bodies 1
extrude "Extrude76" cut 1 faces at (-20.2239, -13, -31.3333) along direction (0, 1, 0) blind 2 on bodies 1 bodies 1
sketch "Sketch40" plane through (0, -18, 0) normal (0, -1, 0) x (1, 0, 0)
  line L0 (32.5, -9.4005) -> (30.75, -9.4005)
  line L1 (30.75, -9.4005) -> (30.75, -30.75)
  line L2 (30.75, -30.75) -> (-15.7732, -30.75)
  line L3 (-15.7732, -30.75) -> (-15.7732, -32.5)
  line L4 (-15.7732, -32.5) -> (27.5, -32.5)
  arc A0 (27.5, -32.5) -> (32.5, -27.5) centre (27.5, -27.5) ccw
  line L5 (32.5, -27.5) -> (32.5, -9.4005)
  line L6 (30.75, -30.75) -> (24.75, -30.75)
  line L7 (24.75, -30.75) -> (12.75, -30.75)
  line L8 (12.75, -30.75) -> (12.75, -32.5)
  line L9 (12.75, -32.5) -> (24.75, -32.5)
  line L10 (24.75, -32.5) -> (24.75, -30.75)
  dimension "d278" = 6
  dimension "d279" = 12
  constraint coincident L1.end L2.start
  constraint perpendicular L1 L6
  constraint horizontal L7
  constraint vertical L8
  constraint horizontal L9
  constraint vertical L10
  measures "d278" distance of L1.end L6.end
  measures "d279" distance of L6.end L7.end
extrude "Extrude77" cut sketch "Sketch40" against normal blind 6 contours L2 L4 L7 L8 L9 L10 bodies 1
copy_body "CopyPasteBodies1" bodies 1 makes body 2
move_body "Move1" bodies 2 to x (1, 0, 0) y (0, 1, 0) z (0, 0, 1) at (-62.6717, -26.7125, 0)
move_body "Move2" bodies 2 to x (1, 0, 0) y (0, 1, 0) z (0, 0, 1) at (-52.218, 25.142, 0)
delete_face "DeleteFace13" 1 faces at (-144.248, -12.9038, -32.1418) on bodies 2
delete_face "DeleteFace14" 1 faces at (-86.9145, -12.9038, -32.4774) on bodies 2
delete_face "DeleteFace15" 1 faces at (-147.2532, -14.2372, 28.6606) on bodies 2
delete_face "DeleteFace16" 1 faces at (-82.5263, -14.2372, 28.6606) on bodies 2
extrude "Extrude78" add 1 faces at (-102.9414, -2.4639, 32.5) along direction (0, 0, 1) blind 2 on bodies 2 bodies 2
extrude "Extrude79" add 1 faces at (-82.3897, -8.5705, -24.8002) along direction (1, 0, 0) blind 2 on bodies 2 bodies 2
extrude "Extrude80" add 1 faces at (-92.0455, -4.9038, -32.5) along direction (0, 0, -1) blind 2 on bodies 2 bodies 2
extrude "Extrude81" add 1 faces at (-147.3897, -8.9038, -27.7856) along direction (-1, 0, 0) blind 2 on bodies 2 bodies 2
sketch "Sketch41" plane through (0, -19.5705, 0) normal (0, -1, 0) x (1, 0, 0)
  line L0 (-149.3897, 23.7576) -> (-145.6397, 23.7576)
  line L1 (-145.6397, 23.7576) -> (-145.6397, 30.75)
  line L2 (-145.6397, 30.75) -> (-84.1397, 30.75)
  line L3 (-84.1397, 30.75) -> (-84.1397, 2.1041)
  line L4 (-84.1397, 2.1041) -> (-80.3897, 2.1041)
  line L5 (-80.3897, 2.1041) -> (-80.3897, 34.5)
  line L6 (-80.3897, 34.5) -> (-149.3897, 34.5)
  line L7 (-149.3897, 34.5) -> (-149.3897, 23.7576)
  line L8 (-149.3897, 34.5) -> (-80.3897, 34.5)
  line L9 (-80.3897, 34.5) -> (-80.3897, 32.9)
  line L10 (-80.3897, 32.9) -> (-149.3897, 32.9)
  line L11 (-149.3897, 32.9) -> (-149.3897, 34.5)
  line L12 (-80.3897, 34.5) -> (-81.9897, 34.5)
  line L13 (-81.9897, 34.5) -> (-81.9897, 2.1041)
  line L14 (-81.9897, 2.1041) -> (-80.3897, 2.1041)
  line L15 (-80.3897, 2.1041) -> (-80.3897, 34.5)
  line L16 (-149.3897, 34.5) -> (-147.7897, 34.5)
  line L17 (-147.7897, 34.5) -> (-147.7897, 23.6687)
  line L18 (-147.7897, 23.6687) -> (-149.3897, 23.6687)
  line L19 (-149.3897, 23.6687) -> (-149.3897, 34.5)
  dimension "d290" = 1.6
  dimension "d291" = 1.6
  dimension "d292" = 1.6
  constraint horizontal L8
  constraint vertical L9
  constraint horizontal L10
  constraint vertical L11
  constraint coincident L6.end L7.start
  constraint horizontal L12
  constraint vertical L13
  constraint horizontal L14
  constraint vertical L15
  constraint horizontal L16
  constraint vertical L17
  constraint horizontal L18
  constraint vertical L19
  measures "d290" distance of L6.end L10.end
  measures "d291" distance of L5.end L12.end
  measures "d292" distance of L6.end L16.end
extrude "Extrude82" add sketch "Sketch41" along normal blind 5 contours L0 L7 L10 L17 L19 | L6 L7 L8 L10 L11 L16 L17 L19 | L6 L8 L10 L13 L17 | L5 L6 L8 L9 L10 L12 L13 L15 | L4 L5 L10 L13 L14 L15 bodies 2
sketch "Sketch42" plane through (0, -19.5705, 0) normal (0, -1, 0) x (1, 0, 0)
  line L0 (-80.3897, -9.4005) -> (-84.1397, -9.4005)
  line L1 (-84.1397, -9.4005) -> (-84.1397, -30.75)
  line L2 (-84.1397, -30.75) -> (-90.1397, -30.75)
  line L3 (-90.1397, -30.75) -> (-90.1397, -34.5)
  line L4 (-90.1397, -34.5) -> (-80.3897, -34.5)
  line L5 (-80.3897, -34.5) -> (-80.3897, -9.4005)
  line L6 (-80.3897, -34.5) -> (-81.9897, -34.5)
  line L7 (-81.9897, -34.5) -> (-81.9897, -9.4005)
  line L8 (-81.9897, -9.4005) -> (-80.3897, -9.4005)
  line L9 (-80.3897, -9.4005) -> (-80.3897, -34.5)
  line L10 (-80.3897, -34.5) -> (-90.1397, -34.5)
  line L11 (-90.1397, -34.5) -> (-90.1397, -32.9)
  line L12 (-90.1397, -32.9) -> (-80.3897, -32.9)
  line L13 (-80.3897, -32.9) -> (-80.3897, -34.5)
  dimension "d295" = 1.6
  dimension "d296" = 1.6
  constraint horizontal L6
  constraint vertical L7
  constraint horizontal L8
  constraint vertical L9
  constraint coincident L4.end L5.start
  constraint horizontal L10
  constraint vertical L11
  constraint horizontal L12
  constraint vertical L13
  measures "d295" distance of L4.end L6.end
  measures "d296" distance of L4.end L12.end
extrude "Extrude83" add sketch "Sketch42" along normal blind 5 contours L0 L5 L7 L8 L9 L12 | L4 L5 L6 L7 L9 L10 L12 L13 | L3 L4 L7 L10 L11 L12 bodies 2
sketch "Sketch43" plane through (0, -19.5705, 0) normal (0, -1, 0) x (1, 0, 0)
  line L0 (-102.1397, -34.5) -> (-102.1397, -30.75)
  line L1 (-102.1397, -30.75) -> (-130.663, -30.75)
  line L2 (-130.663, -30.75) -> (-130.663, -34.5)
  line L3 (-130.663, -34.5) -> (-102.1397, -34.5)
  line L4 (-130.663, -34.5) -> (-102.1397, -34.5)
  line L5 (-102.1397, -34.5) -> (-102.1397, -32.9)
  line L6 (-102.1397, -32.9) -> (-130.663, -32.9)
  line L7 (-130.663, -32.9) -> (-130.663, -34.5)
  dimension "d299" = 1.6
  constraint horizontal L4
  constraint vertical L5
  constraint horizontal L6
  constraint vertical L7
  constraint coincident L2.end L3.start
  measures "d299" distance of L2.end L6.end
extrude "Extrude84" add sketch "Sketch43" along normal blind 5 contours L0 L2 L3 L4 L5 L6 L7 bodies 2
sketch "Sketch44" plane through (0, -19.5705, 0) normal (0, -1, 0) x (1, 0, 0)
  line L0 (-137.339, -34.5) -> (-137.339, -30.75)
  line L1 (-137.339, -30.75) -> (-145.6397, -30.75)
  line L2 (-145.6397, -30.75) -> (-145.6397, -14.3569)
  line L3 (-145.6397, -14.3569) -> (-149.3897, -14.3569)
  line L4 (-149.3897, -14.3569) -> (-149.3897, -34.5)
  line L5 (-149.3897, -34.5) -> (-137.339, -34.5)
  line L6 (-149.3897, -14.3569) -> (-147.7897, -14.3569)
  line L7 (-147.7897, -14.3569) -> (-147.7897, -34.5)
  line L8 (-147.7897, -34.5) -> (-149.3897, -34.5)
  line L9 (-149.3897, -34.5) -> (-149.3897, -14.3569)
  line L10 (-149.3897, -34.5) -> (-137.339, -34.5)
  line L11 (-137.339, -34.5) -> (-137.339, -32.9)
  line L12 (-137.339, -32.9) -> (-149.3897, -32.9)
  line L13 (-149.3897, -32.9) -> (-149.3897, -34.5)
  dimension "d302" = 1.6
  dimension "d303" = 1.6
  constraint horizontal L6
  constraint vertical L7
  constraint horizontal L8
  constraint vertical L9
  constraint coincident L3.end L4.start
  constraint horizontal L10
  constraint vertical L11
  constraint horizontal L12
  constraint vertical L13
  measures "d302" distance of L3.end L6.end
  measures "d303" distance of L4.end L12.end
extrude "Extrude85" add sketch "Sketch44" along normal blind 5 contours L0 L5 L7 L10 L11 L12 | L4 L5 L7 L8 L9 L10 L12 L13 | L3 L4 L6 L7 L9 L12 bodies 2
fillet "Fillet14" radius 5 4 edges at (-80.3897, -20.5705, 34.5) (-149.3897, -20.5705, 34.5) (-80.3897, -12.0705, -34.5) (-149.3897, -12.0705, -34.5) on bodies 2
extrude "Extrude86" cut 1 faces at (-31.3333, -16.5, 23.7576) along direction (0, 0, 1) blind 0.3 on bodies 1 bodies 1
extrude "Extrude87" cut 1 faces at (-32.2333, -14, -3.7173) along direction (0, 0, -1) blind 0.3 on bodies 1 bodies 1
extrude "Extrude88" cut 1 faces at (-31.3333, -17.5, 12.1529) along direction (0, 1, 0) blind 0.4 on bodies 1 bodies 1
extrude "Extrude89" add 1 faces at (-32.1, -10, -7.4115) along direction (1, 0, 0) blind 0.1 on bodies 1 bodies 1
extrude "Extrude90" add 1 faces at (-32.1, -15, 7.7247) along direction (1, 0, 0) blind 0.12 on bodies 1 bodies 1
extrude "Extrude91" add 1 faces at (-32.1, -15, 20.9517) along direction (1, 0, 0) blind 0.1 on bodies 1 bodies 1
extrude "Extrude92" cut 1 faces at (-32.1533, -18, 5.0728) along direction (0, 1, 0) blind 0.8 on bodies 1 bodies 1
extrude "Extrude93" cut 1 faces at (-32.3333, -18, 18.3236) along direction (0, 1, 0) blind 0.8 on bodies 1 bodies 1
extrude "Extrude94" cut 1 faces at (-20.2239, -11, -31.3333) along direction (0, 1, 0) blind 1 on bodies 1 bodies 1
extrude "Extrude95" add 1 faces at (12.75, -16, -31.3333) along direction (1, 0, 0) blind 0.2 on bodies 1 bodies 1
extrude "Extrude96" add 1 faces at (16.8833, -12, -31.3333) along direction (0, -1, 0) blind 0.3 on bodies 1 bodies 1
extrude "Extrude97" cut 1 faces at (-31.3333, -17.1, 12.1529) along direction (0, 1, 0) blind 0.5 on bodies 1 bodies 1
extrude "Extrude98" cut 2 faces at (-32.3333, -17.2, 18.3236) (-32.1533, -17.2, 5.0728) along direction (0, 1, 0) blind 0.5 on bodies 1 bodies 1
extrude "Extrude99" cut 1 faces at (-31.3333, -16.5, 24.0576) along direction (0, 0, 1) blind 0.3 on bodies 1 bodies 1
extrude "Extrude100" cut 1 faces at (-31.9167, -16.5, 2.2148) along direction (0, 0, -1) blind 0.2 on bodies 1 bodies 1
extrude "Extrude101" add 1 faces at (-32.3267, -14.5667, 2.4209) along direction (0, 0, -1) blind 0.2 on bodies 1 bodies 1
extrude "Extrude102" add 1 faces at (-32.3333, -14.5667, 23.5798) along direction (0, 0, 1) blind 0.3 on bodies 1 bodies 1
extrude "Extrude103" add 1 faces at (12.95, -14.2, -31.3333) along direction (1, 0, 0) blind 1 on bodies 1 bodies 1
sketch "Sketch45" plane through (24.75, 0, 0) normal (-1, 0, 0) x (0, 0, 1)
  line L0 (-30.75, -12.3) -> (-32.5, -12.3)
  line L1 (-32.5, -12.3) -> (-32.5, -18)
  line L2 (-32.5, -18) -> (-30.75, -18)
  line L3 (-30.75, -18) -> (-30.75, -13)
  line L4 (-30.75, -13) -> (-28.75, -13)
  line L5 (-28.75, -13) -> (-28.75, 0)
  line L6 (-28.75, 0) -> (-30.75, 0)
  line L7 (-30.75, 0) -> (-30.75, -12.3)
  line L8 (-32.5, -12.3) -> (-30.75, -12.3)
  line L9 (-30.75, -12.3) -> (-30.75, -18)
  line L10 (-30.75, -18) -> (-32.5, -18)
  line L11 (-32.5, -18) -> (-32.5, -12.3)
  constraint horizontal L8
  constraint vertical L9
  constraint horizontal L10
  constraint vertical L11
  constraint coincident L2.end L3.start
  constraint coincident L0.end L1.start
extrude "Extrude104" add sketch "Sketch45" along normal blind 1 contours L0 L1 L2 L3 L8 L9 L10 L11 bodies 1
hidden bodies 2
equation "d232 = 0 mm - 0.5 mm"
named bodies: "Com_Top_A", "Com_Top_A (1)"
